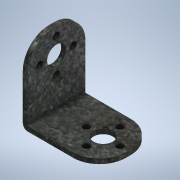
# Autodesk Inventor part: уголок
Saved by Autodesk Inventor 2020.1 (Build 241239000, 239)
## iProperties
Created: 2021-08-18
Part Number: уголок
Material: Сталь
Document SubType Name: Modeling
Designer: User
Density: 7.85 g/cm^3
Appearance: Листовая
Author: User
Autodesk Inventor part; units mm, degrees
ref_plane "YZ Plane" through (0, 0, 0) normal (1, 0, 0) x (0, 1, 0)
ref_plane "XZ Plane" through (0, 0, 0) normal (0, 1, 0) x (-1, 0, 0)
ref_plane "XY Plane" through (0, 0, 0) normal (0, 0, 1) x (1, 0, 0)
sketch "Эскиз1" plane through (0, 0, 0) normal (0, 1, 0) x (-1, 0, 0)
  line L0 (15.0734, 10.2239) -> (-16.9266, 10.2239)
  line L1 (-16.9266, 10.2239) -> (-16.9266, -13.7761)
  line L2 (-16.9266, -13.7761) -> (15.0734, -13.7761)
  line L3 (15.0734, -13.7761) -> (15.0734, 10.2239)
  point P0 (0, 0)
  dimension "d0" = 32
  dimension "d1" = 24
  constraints: 8 end point, 2 parallel, 1 horizontal, 1 perpendicular
  measures "d0" distance of L1.end L2.end
  measures "d1" distance of L1.end L0.end
extrude "Выдавливание1" add sketch "Эскиз1" along normal blind 2
sketch "Эскиз2" plane through (0, 2, 0) normal (0, 1, 0) x (1, 0, 0)
  line L0 (16.9266, 13.7761) -> (-15.0734, 13.7761) projected
  line L1 (-15.0734, -10.2239) -> (16.9266, -10.2239) projected
  line L2 (-15.0734, 13.7761) -> (-13.0734, 13.7761)
  line L3 (-13.0734, 13.7761) -> (-13.0734, -10.2239)
  line L4 (-13.0734, -10.2239) -> (-15.0734, -10.2239)
  line L5 (-15.0734, -10.2239) -> (-15.0734, 13.7761)
  point P0 (0, 0)
  dimension "d4" = 2
  constraints: 8 end point, 2 parallel, 1 horizontal, 1 perpendicular, 1 point on line
  measures "d4" distance of L3.end L4.end
extrude "Выдавливание2" add sketch "Эскиз2" along normal blind 30
sketch "Эскиз3" plane through (-13.0734, 2, 10.2239) normal (1, 0, 0) x (0, 0, -1)
  circle A0 centre (12, 19.5) radius 4
  circle A1 centre (12, 19.5) radius 7
  line L0 (24, 30) -> (0, 30) projected
  line L1 (24, 0) -> (24, 30) projected
  circle A2 centre (19, 19.5) radius 1.5
  circle A3 centre (12, 12.5) radius 1.5
  circle A4 centre (5, 19.5) radius 1.5
  circle A5 centre (12, 26.5) radius 1.5
  point P0 (10.2239, -2)
  point P1 (12, 30)
  dimension "d7" = 8
  dimension "d8" = 14
  dimension "d10" = 12
  dimension "d11" = 3
  dimension "d12" = 3
  dimension "d13" = 3
  dimension "d14" = 3
  dimension "d15" = 3.5
  dimension "d16" = 0
  dimension "d17" = 0
  dimension "d18" = 0
  dimension "d19" = 7
  constraints: 6 centre point, 3 point on circle, 1 coincident, 1 midpoint
  measures "d7" diameter of A0
  measures "d8" diameter of A1
  measures "d10" distance from line of L1 A0.centre
  measures "d11" diameter of A2
  measures "d12" diameter of A3
  measures "d13" diameter of A4
  measures "d14" diameter of A5
  measures "d15" distance of A5.centre point (12, 30)
  measures "d16" vertical distance of A0.centre A4.centre
  measures "d17" vertical distance of A2.centre A0.centre
  measures "d18" horizontal distance of A3.centre A0.centre
  measures "d19" distance of A0.centre A4.centre
extrude "Выдавливание3" cut sketch "Эскиз3" against normal blind 100 contours A0 | A1 A2 | A1 A2 | A5 A1 | A1 A5 | A3 A1 | A1 A3 | A4 A1 | A1 A4
sketch "Эскиз4" plane through (0, 2, 0) normal (0, 1, 0) x (1, 0, 0)
  circle A0 centre (6.4266, 1.7761) radius 4
  circle A1 centre (6.4266, 1.7761) radius 7
  circle A2 centre (6.4266, -5.2239) radius 1.5
  circle A3 centre (6.4266, 8.7761) radius 1.5
  circle A4 centre (-0.5734, 1.7761) radius 1.5
  circle A5 centre (13.4266, 1.7761) radius 1.5
  line L0 (16.9266, -10.2239) -> (16.9266, 13.7761) projected
  line L1 (16.9266, 13.7761) -> (-13.0734, 13.7761) projected
  point P0 (0, 0)
  point P1 (16.9266, 1.7761)
  dimension "d22" = 8
  dimension "d23" = 14
  dimension "d24" = 3
  dimension "d25" = 3
  dimension "d26" = 3
  dimension "d27" = 3
  dimension "d29" = 12
  dimension "d30" = 3.5
  constraints: 6 centre point, 4 point on circle, 1 coincident, 1 midpoint
  measures "d22" diameter of A0
  measures "d23" diameter of A1
  measures "d24" diameter of A2
  measures "d25" diameter of A3
  measures "d26" diameter of A4
  measures "d27" diameter of A5
  measures "d29" distance from line of L1 A0.centre
  measures "d30" distance from line of L0 A5.centre
extrude "Выдавливание4" cut sketch "Эскиз4" against normal blind 100 contours A0 | A1 A5 | A1 A5 | A3 A1 | A1 A3 | A2 A1 | A1 A2 | A4 A1 | A1 A4
fillet "Сопряжение1" radius 11 4 edges at (-14.0734, 32, 10.2239) (-14.0734, 32, -13.7761) (16.9266, 1, -13.7761) (16.9266, 1, 10.2239)
fillet "Сопряжение2" radius 2 1 edges at (-15.0734, 0, -1.7761)
